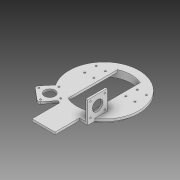
# Autodesk Inventor part: SwivelMount
Saved by Autodesk Inventor 2020 (Build 240168000, 168)
## iProperties
Created: 2020-09-15
Part Number: SwivelMount
Material: Generic
Document SubType Name: Modeling
Designer: DDeGo
Density: 1 g/cm^3
Appearance: Default
Author: DDeGo
Autodesk Inventor part; units mm, degrees
ref_plane "YZ Plane" through (0, 0, 0) normal (1, 0, 0) x (0, 1, 0)
ref_plane "XZ Plane" through (0, 0, 0) normal (0, 1, 0) x (-1, 0, 0)
ref_plane "XY Plane" through (0, 0, 0) normal (0, 0, 1) x (1, 0, 0)
sketch "Sketch1" plane through (0, 0, 0) normal (1, 0, 0) x (0, 1, 0)
  line L0 (0, 0) -> (0, -59.4) construction
  line L1 (0, -59.4) -> (7.5, -59.4)
  line L2 (7.5, -59.4) -> (7.5, -66.4) construction
  line L3 (7.5, -66.4) -> (5, -66.4)
  line L4 (5, -66.4) -> (5, -63.4)
  line L5 (5, -63.4) -> (0, -63.4)
  line L6 (0, -63.4) -> (0, -59.4)
  line L7 (0, 0) -> (7.5, 0) construction
  line L8 (7.5, 0) -> (7.5, -66.4) construction
  line L9 (7.5, -66.4) -> (11, -66.4)
  line L10 (11, -66.4) -> (11, -76)
  line L11 (11, -76) -> (16, -76)
  line L12 (16, -76) -> (16, -59.4)
  line L13 (16, -59.4) -> (7.5, -59.4)
  dimension "d0" = 63.4
  dimension "d1" = 4
  dimension "d2" = 2.5
  dimension "d3" = 3
  dimension "d4" = 5
  dimension "d6" = 6
  dimension "d7" = 5
  dimension "d8" = 76
  constraints: 28 end point, 10 perpendicular, 2 horizontal, 1 collinear, 1 point on line, 1 vertical
  measures "d0" distance from line of L0.start L5
  measures "d1" distance between parallel lines of L1 L5
  measures "d2" distance between parallel lines of L2 L4
  measures "d3" distance of L3.end L4.end
  measures "d4" distance of L4.end L5.end
  measures "d6" distance between parallel lines of L4 L10
  measures "d7" distance of L10.end L11.end
  measures "d8" distance between parallel lines of L7 L11
revolve "Revolution1" add sketch "Sketch1" angle 360 about axis through (0, 0, 0) along (0, 1, 0)
sketch "Sketch2" plane through (0, 16, 0) normal (0, 1, 0) x (1, 0, 0)
  line L0 (-24.75, -59.4) -> (24.75, -59.4)
  line L1 (24.75, -59.4) -> (24.75, 59.4)
  line L2 (24.75, 59.4) -> (-24.75, 59.4)
  line L3 (-24.75, 59.4) -> (-24.75, -59.4)
  line L4 (-24.75, -59.4) -> (24.75, 59.4) construction
  line L5 (24.75, -59.4) -> (-24.75, 59.4) construction
  circle A0 centre (0, 0) radius 59.4 projected
  point P0 (24.75, -53.9981)
  point P1 (24.75, 53.9981)
  point P2 (-24.75, -53.9981)
  point P3 (-24.75, 53.9981)
  dimension "d9" = 49.5
  constraints: 12 end point, 2 midpoint, 2 parallel, 1 horizontal, 1 perpendicular, 1 tangent
  measures "d9" distance of L1.end L2.end
extrude "Extrusion1" add sketch "Sketch2" against normal blind 5 contours A0 L3 | L1 A0
sketch "Sketch3" plane through (0, 16, 0) normal (0, 1, 0) x (1, 0, 0)
  line L0 (-44.75, 25) -> (0, 25) construction
  line L1 (24.75, 53.9981) -> (24.75, -53.9981) projected
  line L2 (-24.75, -53.9981) -> (-24.75, 53.9981) projected
  line L3 (-34.75, 12.5) -> (-54.75, 12.5) construction
  line L4 (-54.75, 12.5) -> (-54.75, 37.5) construction
  line L5 (-54.75, 37.5) -> (-34.75, 37.5) construction
  line L6 (-34.75, 37.5) -> (-34.75, 12.5) construction
  line L7 (-34.75, 12.5) -> (-54.75, 37.5) construction
  line L8 (-54.75, 12.5) -> (-34.75, 37.5) construction
  line L9 (0, 0) -> (0, 25) construction
  circle A0 centre (-54.75, 12.5) radius 1.75
  circle A1 centre (-54.75, 37.5) radius 1.75
  circle A2 centre (-34.75, 37.5) radius 1.75
  circle A3 centre (-34.75, 12.5) radius 1.75
  line L10 (34.75, 12.5) -> (54.75, 12.5) construction
  line L11 (54.75, 12.5) -> (54.75, 37.5) construction
  line L12 (54.75, 37.5) -> (34.75, 37.5) construction
  line L13 (34.75, 37.5) -> (34.75, 12.5) construction
  line L14 (34.75, 12.5) -> (54.75, 37.5) construction
  line L15 (54.75, 12.5) -> (34.75, 37.5) construction
  circle A4 centre (54.75, 12.5) radius 1.75
  circle A5 centre (54.75, 37.5) radius 1.75
  circle A6 centre (34.75, 37.5) radius 1.75
  circle A7 centre (34.75, 12.5) radius 1.75
  point P0 (44.75, 25)
  dimension "d12" = 25
  dimension "d14" = 20
  dimension "d15" = 25
  dimension "d16" = 20
  dimension "d17" = 3.5
  constraints: 28 end point, 9 symmetric about line, 8 centre point, 8 coincident, 4 midpoint, 3 equal radius, 2 horizontal, 2 parallel, 1 perpendicular, 1 vertical, 4 other
  measures "d12" distance from line of L9.start L0
  measures "d14" distance from line of L0.start L2
  measures "d15" distance of L3.end L4.end
  measures "d16" distance of L4.end L5.end
  measures "d17" diameter of A0
extrude "Extrusion2" cut sketch "Sketch3" against normal through all
sketch "Sketch4" plane through (0, 16, 0) normal (0, 1, 0) x (1, 0, 0)
  circle A0 centre (0, 0) radius 76 projected
  line L0 (25, -131.7705) -> (-25, -131.7705)
  line L1 (-25, -131.7705) -> (-25, -71.7705)
  line L2 (-25, -71.7705) -> (25, -71.7705) construction
  line L3 (25, -71.7705) -> (25, -131.7705)
  line L4 (25, -131.7705) -> (-25, -71.7705) construction
  line L5 (-25, -131.7705) -> (25, -71.7705) construction
  line L6 (0, -101.7705) -> (0, 0) construction
  point P0 (0, 0)
  dimension "d20" = 60
  dimension "d21" = 50
  constraints: 14 end point, 2 midpoint, 2 parallel, 1 horizontal, 1 perpendicular, 1 vertical, 2 other
  measures "d20" distance of L0.end L1.end
  measures "d21" distance of L0.start L0.end
extrude "Extrusion3" add sketch "Sketch4" against normal up to surface (5 mm away) contours A0 L3 L0 L1
sketch "Sketch5" plane through (-25, 16, 131.7705) normal (0, 1, 0) x (1, 0, 0)
  line L0 (-31.5826, 97.0082) -> (0.5913, 70.0111)
  line L1 (0.5913, 70.0111) -> (-23.1918, 41.6675)
  line L2 (-30.236, 41.0512) -> (-54.7494, 61.6204)
  line L3 (-55.3657, 68.6646) -> (-31.5826, 97.0082)
  line L4 (-7.1573, 69.3332) -> (-30.9046, 89.2596) construction
  line L5 (-30.9046, 89.2596) -> (-50.8311, 65.5123) construction
  line L6 (-50.8311, 65.5123) -> (-27.0837, 45.5858) construction
  line L7 (-27.0837, 45.5858) -> (-7.1573, 69.3332) construction
  arc A0 (50, 60) -> (0, 60) centre (25, 131.7705) ccw projected
  line L8 (-50.8311, 65.5123) -> (-7.1573, 69.3332) construction
  circle A1 centre (25, 131.7705) radius 63.4 projected
  line L9 (-28.9942, 67.4227) -> (-15.7527, 83.2032) construction
  line L10 (-15.7527, 83.2032) -> (25, 131.7705) construction
  circle A2 centre (-30.9046, 89.2596) radius 1.75
  circle A3 centre (-50.8311, 65.5123) radius 1.75
  circle A4 centre (-28.9942, 67.4227) radius 11.5
  circle A5 centre (-27.0837, 45.5858) radius 1.75
  circle A6 centre (-7.1573, 69.3332) radius 1.75
  line L11 (25, 131.7705) -> (25, 92.5102) construction
  arc A7 (-55.3657, 68.6646) -> (-54.7494, 61.6204) centre (-51.5355, 65.4506) ccw
  arc A8 (-30.236, 41.0512) -> (-23.1918, 41.6675) centre (-27.022, 44.8814) ccw
  point P0 (-26.4058, 37.8373)
  point P1 (-58.5796, 64.8343)
  point P2 (-5.863, 62.3192)
  point P3 (-38.0368, 89.3163)
  dimension "d24" = 20.6
  dimension "d25" = 31
  dimension "d26" = 42
  dimension "d29" = 3.5
  dimension "d30" = 23
  dimension "d31" = 40
  dimension "d37" = 5
  dimension "d38" = 84
  constraints: 24 end point, 7 centre point, 5 coincident, 4 equal radius, 4 parallel, 4 perpendicular, 4 point on circle, 4 point on line, 4 tangent, 1 collinear, 1 midpoint, 1 vertical, 5 other
  measures "d24" distance of L9.start L9.end
  measures "d25" distance of L5.end L6.end
  measures "d26" distance of point (-26.406, 37.837) point (-58.58, 64.834)
  measures "d29" diameter of A6
  measures "d30" diameter of A4
  measures "d31" angle of L10 L11
  measures "d37" radius of A7
  measures "d38" distance of point (25, 131.77) A4.centre
extrude "Extrusion4" add sketch "Sketch5" against normal up to surface (5 mm away) contours L0 A1 L1 A0 A4 L3 | L0 A1 | A0 A4 L1 A8 L2 A7 L3 | A4 A0 | A0 A4 | A2 | A3 | A5 | A6 picked at (-14.9655, 82.9101)
extrude "Extrusion5" cut sketch "Sketch5" against normal through all contours A4 A0 | A0 A4 | A2 | A3 | A5 | A6
sketch "Sketch6" plane through (-25, 11, 131.7705) normal (0, -1, 0) x (1, 0, 0)
  circle A0 centre (-50.8311, -65.5123) radius 1.75 projected
  circle A1 centre (-50.8311, -65.5123) radius 3
  circle A2 centre (-27.0837, -45.5858) radius 1.75 projected
  circle A3 centre (-27.0837, -45.5858) radius 3
  circle A4 centre (-7.1573, -69.3332) radius 1.75 projected
  circle A5 centre (-7.1573, -69.3332) radius 3
  circle A6 centre (-30.9046, -89.2596) radius 1.75 projected
  circle A7 centre (-30.9046, -89.2596) radius 3
  point P0 (25, -131.7705)
  dimension "d34" = 6
  constraints: 4 centre point, 4 coincident, 3 equal radius
  measures "d34" diameter of A1
extrude "Extrusion6" cut sketch "Sketch6" against normal blind 3 contours A0 | A1 | A2 | A3 | A4 | A5 | A6 | A7
ref_plane "Work Plane1" through (38.75, 16, -53.9981) normal (-1, 0, 0) x (0, 0, 1)
sketch "Sketch7" plane through (38.75, 16, -53.9981) normal (-1, 0, 0) x (0, 0, 1)
  line L0 (14.7481, 0) -> (18.2481, 0) projected
  line L1 (39.7481, 0) -> (43.2481, 0) projected
  line L2 (16.4981, 0) -> (28.9981, 40) construction
  line L3 (28.9981, 40) -> (41.4981, 0) construction
  line L4 (28.9981, 40) -> (110.9356, 21.5) construction
  line L5 (95.4356, 37) -> (126.4356, 37) construction
  line L6 (126.4356, 37) -> (126.4356, 6) construction
  line L7 (126.4356, 6) -> (95.4356, 6) construction
  line L8 (95.4356, 6) -> (95.4356, 37) construction
  line L9 (95.4356, 37) -> (126.4356, 6) construction
  line L10 (126.4356, 37) -> (95.4356, 6) construction
  circle A0 centre (110.9356, 21.5) radius 11.5
  circle A1 centre (126.4356, 37) radius 1.75
  circle A2 centre (126.4356, 6) radius 1.75
  circle A3 centre (95.4356, 6) radius 1.75
  circle A4 centre (95.4356, 37) radius 1.75
  line L11 (89.4356, 0) -> (132.4356, 0)
  line L12 (132.4356, 0) -> (132.4356, 43)
  line L13 (132.4356, 43) -> (89.4356, 43)
  line L14 (89.4356, 43) -> (89.4356, 0)
  line L15 (89.4356, 0) -> (132.4356, 43) construction
  line L16 (132.4356, 0) -> (89.4356, 43) construction
  line L17 (0, 0) -> (107.9962, 0) projected
  point P0 (53.9981, -16)
  dimension "d40" = 84
  dimension "d41" = 23
  dimension "d42" = 3.5
  dimension "d43" = 31
  dimension "d44" = 31
  dimension "d46" = 40
  dimension "d47" = 43
  constraints: 30 end point, 6 midpoint, 5 centre point, 5 coincident, 4 parallel, 3 equal radius, 2 horizontal, 2 perpendicular, 1 equal length, 1 point on line, 2 other
  measures "d40" distance of L2.end L4.end
  measures "d41" diameter of A0
  measures "d42" diameter of A4
  measures "d43" distance of L5.start L5.end
  measures "d44" distance of L7.end L5.start
  measures "d46" distance from line of L1 L2.end
  measures "d47" distance of L11.end L12.end
extrude "Extrusion7" add sketch "Sketch7" against normal blind 4
sketch "Sketch8" plane through (38.75, 16, 65.3792) normal (0, -1, 0) x (1, 0, 0)
  arc A0 (-101.7868, -22.925) -> (4, -2.5426) centre (-38.75, -65.3792) ccw projected
  line L0 (0, 13.0583) -> (4, 13.0583) projected
  line L1 (4, -2.5426) -> (4, 13.0583)
  line L2 (4, 13.0583) -> (-13.75, 13.0583)
  line L3 (-13.75, 66.3913) -> (-13.75, 6.3913) projected
  arc A1 (0, 0) -> (-13.75, 6.3913) centre (-38.75, -65.3792) ccw projected
  line L4 (-13.75, 13.0583) -> (-13.75, 6.3913)
  arc A2 (4, -2.5426) -> (-13.75, 6.3913) centre (-38.75, -65.3792) ccw
  arc A3 (-101.7868, -22.925) -> (-13.75, 6.3913) centre (-38.75, -65.3792) ccw projected
  constraints: 6 end point, 2 perpendicular, 2 point on circle, 1 centre point, 1 concentric, 1 point on line, 1 vertical
extrude "Extrusion8" add sketch "Sketch8" along normal up to surface (5 mm away)
body "Solid1"
